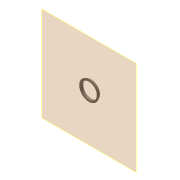
# Autodesk Inventor part: 30_Cube_Insert_Filter_Revolver_Wheel_centerring_v3
Saved by Autodesk Inventor 2019.4 (Build 234330000, 330)
## iProperties
Created: 2021-09-14
Part Number: 30_Cube_Insert_Filter_Revolver_Wheel_centerring_v3
Material: Generic
Document SubType Name: Modeling
Designer: diederichbenedict
Density: 1 g/cm^3
Appearance: Default
Author: diederichbenedict
Autodesk Inventor part; units mm, degrees
ref_plane "YZ Plane" through (0, 0, 0) normal (1, 0, 0) x (0, 1, 0)
ref_plane "XZ Plane" through (0, 0, 0) normal (0, 1, 0) x (-1, 0, 0)
ref_plane "XY Plane" through (0, 0, 0) normal (0, 0, 1) x (1, 0, 0)
ref_plane "Work Plane1" through (0, 0, 0) normal (0, 0, 1) x (1, 0, 0)
sketch "Sketch1" plane through (0, 0, 0) normal (0, 0, 1) x (1, 0, 0)
  circle A0 centre (0, 0) radius 10 projected
  line L0 (-7.2, -1.1879) -> (-7.2, -4.5729) projected
  line L1 (-7.0536, -4.9264) -> (-4.9264, -7.0536) projected
  line L2 (-4.5729, -7.2) -> (-1.1879, -7.2) projected
  circle A1 centre (0, 0) radius 8.8981
  point P0 (0, 0)
  constraints: 1 centre point
extrude "Extrusion1" add sketch "Sketch1" against normal blind 2.5 draft -1
sketch "Sketch2" plane through (0, 0, 0) normal (0, 0, -1) x (-1, 0, 0)
  line L0 (-43.3828, 4.8719) -> (-44.2046, 1.8046) projected
  line L1 (-44.2046, 1.8046) -> (-47.2719, 0.9828) projected
  line L2 (-47.2719, 0.9828) -> (-49.5172, 3.2281) projected
  line L3 (-49.5172, 3.2281) -> (-48.6954, 6.2954) projected
  line L4 (-48.6954, 6.2954) -> (-45.6281, 7.1172) projected
  line L5 (-45.6281, 7.1172) -> (-43.3828, 4.8719) projected
  line L6 (-3.2281, 49.5172) -> (-0.9828, 47.2719) projected
  line L7 (-0.9828, 47.2719) -> (-1.8046, 44.2046) projected
  line L8 (-1.8046, 44.2046) -> (-4.8719, 43.3828) projected
  line L9 (-4.8719, 43.3828) -> (-7.1172, 45.6281) projected
  line L10 (-7.1172, 45.6281) -> (-6.2954, 48.6954) projected
  line L11 (-6.2954, 48.6954) -> (-3.2281, 49.5172) projected
  circle A0 centre (-10.95, 4.59) radius 2.475 projected
  circle A1 centre (-45.91, 10.95) radius 2.475 projected
  circle A2 centre (-39.55, 45.91) radius 2.475 projected
  circle A3 centre (-4.59, 39.55) radius 2.475 projected
  circle A4 centre (-4.59, 10.95) radius 2.475 projected
  circle A5 centre (-10.95, 45.91) radius 2.475 projected
  circle A6 centre (-45.91, 39.55) radius 2.475 projected
  circle A7 centre (-39.55, 4.59) radius 2.475 projected
  arc A8 (-44.21, 34.05) -> (-47.61, 34.05) centre (-45.91, 34.05) ccw projected
  line L12 (-44.21, 34.05) -> (-44.21, 16.45) projected
  arc A9 (-47.61, 16.45) -> (-44.21, 16.45) centre (-45.91, 16.45) ccw projected
  line L13 (-47.61, 16.45) -> (-47.61, 34.05) projected
  arc A10 (-2.89, 34.05) -> (-6.29, 34.05) centre (-4.59, 34.05) ccw projected
  line L14 (-2.89, 34.05) -> (-2.89, 16.45) projected
  arc A11 (-6.29, 16.45) -> (-2.89, 16.45) centre (-4.59, 16.45) ccw projected
  line L15 (-6.29, 16.45) -> (-6.29, 34.05) projected
  arc A12 (-16.45, 44.21) -> (-16.45, 47.61) centre (-16.45, 45.91) ccw projected
  line L16 (-16.45, 44.21) -> (-34.05, 44.21) projected
  arc A13 (-34.05, 47.61) -> (-34.05, 44.21) centre (-34.05, 45.91) ccw projected
  line L17 (-34.05, 47.61) -> (-16.45, 47.61) projected
  arc A14 (-34.05, 6.29) -> (-34.05, 2.89) centre (-34.05, 4.59) ccw projected
  line L18 (-34.05, 6.29) -> (-16.45, 6.29) projected
  arc A15 (-16.45, 2.89) -> (-16.45, 6.29) centre (-16.45, 4.59) ccw projected
  line L19 (-16.45, 2.89) -> (-34.05, 2.89) projected
  line L20 (-42.22, 42.22) -> (-8.28, 42.22) projected
  line L21 (-8.28, 42.22) -> (-8.28, 8.28) projected
  line L22 (-8.28, 8.28) -> (-42.22, 8.28) projected
  line L23 (-42.22, 8.28) -> (-42.22, 42.22) projected
  circle A16 centre (-46.45, 46.45) radius 2.75 projected
  circle A17 centre (-4.05, 4.05) radius 2.75 projected
  arc A18 (-48.1, 49.6) -> (-49.6, 48.1) centre (-48.1, 48.1) ccw projected
  line L24 (-49.6, 2.4) -> (-49.6, 48.1) projected
  arc A19 (-49.6, 2.4) -> (-48.1, 0.9) centre (-48.1, 2.4) ccw projected
  line L25 (-2.4, 0.9) -> (-48.1, 0.9) projected
  arc A20 (-2.4, 0.9) -> (-0.9, 2.4) centre (-2.4, 2.4) ccw projected
  line L26 (-0.9, 48.1) -> (-0.9, 2.4) projected
  arc A21 (-0.9, 48.1) -> (-2.4, 49.6) centre (-2.4, 48.1) ccw projected
  line L27 (-48.1, 49.6) -> (-2.4, 49.6) projected
  circle A22 centre (0, 0) radius 8.9417 projected
  circle A23 centre (0, 0) radius 9.9564 projected
  circle A24 centre (0, 0) radius 10.9888
  point P0 (0, 0)
  constraints: 1 centre point
extrude "Extrusion2" add sketch "Sketch2" along normal blind 0.5 contours A0 A23 | A0 A23 A4 L26 A22 L25 | A23 A0 A24 | A0 A24 A4 A23 | A23 L25 A24 A0 | A23 A4 | A4 A24 A23 | A23 L26 A24 L25 | L25 A22 L26 A23 | A4 A24 L26 A23
body "Solid1"
